Autodesk Fusion 360 part; units mm, degrees
(part 5 of 11)
  line L3350 (-0.0459, -214.2627) -> (-0.0798, -214.2989)
  line L3351 (-0.0798, -214.2989) -> (-0.1133, -214.3397)
  line L3352 (-0.1133, -214.3397) -> (-0.1441, -214.3827)
  line L3353 (-0.1441, -214.3827) -> (-0.172, -214.4275)
  line L3354 (-0.172, -214.4275) -> (-0.1969, -214.4741)
  line L3355 (-0.1969, -214.4741) -> (-0.2187, -214.5222)
  line L3356 (-0.2187, -214.5222) -> (-0.2373, -214.5717)
  line L3357 (-0.2373, -214.5717) -> (-0.2526, -214.6222)
  line L3358 (-0.2526, -214.6222) -> (-0.2646, -214.6736)
  line L3359 (-0.2646, -214.6736) -> (-0.2732, -214.7258)
  line L3360 (-0.2732, -214.7258) -> (-0.2786, -214.7804)
  line L3361 (-0.2786, -214.7804) -> (-0.28, -214.8985)
  line L3362 (-0.28, -214.8985) -> (-0.28, -218.4997)
  line L3363 (-0.28, -218.4997) -> (-0.28, -219.4997)
  arc A210 (-0.28, -219.4997) -> (0.42, -220.1997) centre (0.42, -219.4997) ccw
  line L3364 (0.42, -220.1997) -> (1.42, -220.1997)
  line L3365 (1.42, -220.1997) -> (5.0918, -220.1997)
  line L3366 (5.0918, -220.1997) -> (5.1413, -220.198)
  line L3367 (5.1413, -220.198) -> (5.1939, -220.1929)
  line L3368 (5.1939, -220.1929) -> (5.246, -220.1843)
  line L3369 (5.246, -220.1843) -> (5.2975, -220.1723)
  line L3370 (5.2975, -220.1723) -> (5.348, -220.1569)
  line L3371 (5.348, -220.1569) -> (5.3974, -220.1383)
  line L3372 (5.3974, -220.1383) -> (5.4455, -220.1165)
  line L3373 (5.4455, -220.1165) -> (5.4921, -220.0916)
  line L3374 (5.4921, -220.0916) -> (5.537, -220.0637)
  line L3375 (5.537, -220.0637) -> (5.5799, -220.033)
  line L3376 (5.5799, -220.033) -> (5.6207, -219.9995)
  line L3377 (5.6207, -219.9995) -> (5.6569, -219.9656)
  line L3378 (5.6569, -219.9656) -> (6.94, -218.6825)
  arc A211 (6.94, -218.6825) -> (6.6572, -217.9997) centre (6.6572, -218.3997) ccw
  line L3379 (6.6572, -217.9997) -> (4.62, -217.9997)
  line L3380 (4.62, -217.9997) -> (4.62, -216.6432)
  line L3381 (4.62, -216.6432) -> (7.1635, -214.0997)
  line L3382 (7.1635, -214.0997) -> (9.7981, -214.0997)
  line L3383 (9.7981, -214.0997) -> (9.9208, -213.977)
  line L3384 (9.9208, -213.977) -> (10.0448, -214.0997)
  line L3385 (10.0448, -214.0997) -> (12.6765, -214.0997)
  line L3386 (12.6765, -214.0997) -> (15.22, -216.6432)
  line L3387 (15.22, -216.6432) -> (15.22, -217.9997)
  line L3388 (15.22, -217.9997) -> (13.1828, -217.9997)
  arc A212 (13.1828, -217.9997) -> (12.9, -218.6825) centre (13.1828, -218.3997) ccw
  line L3389 (12.9, -218.6825) -> (14.1831, -219.9656)
  line L3390 (14.1831, -219.9656) -> (14.2193, -219.9995)
  line L3391 (14.2193, -219.9995) -> (14.2601, -220.033)
  line L3392 (14.2601, -220.033) -> (14.303, -220.0637)
  line L3393 (14.303, -220.0637) -> (14.3479, -220.0916)
  line L3394 (14.3479, -220.0916) -> (14.3945, -220.1165)
  line L3395 (14.3945, -220.1165) -> (14.4426, -220.1383)
  line L3396 (14.4426, -220.1383) -> (14.492, -220.1569)
  line L3397 (14.492, -220.1569) -> (14.5425, -220.1723)
  line L3398 (14.5425, -220.1723) -> (14.594, -220.1843)
  line L3399 (14.594, -220.1843) -> (14.6461, -220.1929)
  line L3400 (14.6461, -220.1929) -> (14.6987, -220.198)
  line L3401 (14.6987, -220.198) -> (14.7482, -220.1997)
  line L3402 (14.7482, -220.1997) -> (18.42, -220.1997)
  line L3403 (18.42, -220.1997) -> (19.42, -220.1997)
  arc A213 (19.42, -220.1997) -> (20.12, -219.4997) centre (19.42, -219.4997) ccw
  line L3404 (20.12, -219.4997) -> (20.12, -218.4997)
  line L3405 (20.12, -218.4997) -> (20.12, -214.8278)
  line L3406 (20.12, -214.8278) -> (20.1184, -214.7783)
  line L3407 (20.1184, -214.7783) -> (20.1132, -214.7258)
  line L3408 (20.1132, -214.7258) -> (20.1046, -214.6736)
  line L3409 (20.1046, -214.6736) -> (20.0926, -214.6222)
  line L3410 (20.0926, -214.6222) -> (20.0773, -214.5717)
  line L3411 (20.0773, -214.5717) -> (20.0587, -214.5222)
  line L3412 (20.0587, -214.5222) -> (20.0369, -214.4741)
  line L3413 (20.0369, -214.4741) -> (20.012, -214.4275)
  line L3414 (20.012, -214.4275) -> (19.9841, -214.3827)
  line L3415 (19.9841, -214.3827) -> (19.9533, -214.3397)
  line L3416 (19.9533, -214.3397) -> (19.9198, -214.2989)
  line L3417 (19.9198, -214.2989) -> (19.8859, -214.2627)
  line L3418 (19.8859, -214.2627) -> (18.6028, -212.9797)
  arc A214 (18.6028, -212.9797) -> (17.92, -213.2625) centre (18.32, -213.2625) ccw
  line L3419 (17.92, -213.2625) -> (17.92, -215.2997)
  line L3420 (17.92, -215.2997) -> (16.5635, -215.2997)
  line L3421 (16.5635, -215.2997) -> (14.02, -212.7562)
  line L3422 (14.02, -212.7562) -> (14.02, -210.1167)
  line L3423 (14.02, -210.1167) -> (13.903, -209.9997)
  line L3424 (13.903, -209.9997) -> (14.02, -209.8826)
  line L3425 (14.02, -209.8826) -> (14.02, -207.2432)
  line L3426 (14.02, -207.2432) -> (16.5635, -204.6997)
  line L3427 (16.5635, -204.6997) -> (17.92, -204.6997)
  line L3428 (17.92, -204.6997) -> (17.92, -206.7368)
  arc A215 (17.92, -206.7368) -> (18.6028, -207.0197) centre (18.32, -206.7368) ccw
  line L3429 (18.6028, -207.0197) -> (19.8859, -205.7366)
  line L3430 (19.8859, -205.7366) -> (19.9198, -205.7004)
  line L3431 (19.9198, -205.7004) -> (19.9533, -205.6596)
  line L3432 (19.9533, -205.6596) -> (19.9841, -205.6166)
  line L3433 (19.9841, -205.6166) -> (20.012, -205.5718)
  line L3434 (20.012, -205.5718) -> (20.0369, -205.5252)
  line L3435 (20.0369, -205.5252) -> (20.0587, -205.4771)
  line L3436 (20.0587, -205.4771) -> (20.0773, -205.4277)
  line L3437 (20.0773, -205.4277) -> (20.0926, -205.3771)
  line L3438 (20.0926, -205.3771) -> (20.1046, -205.3257)
  line L3439 (20.1046, -205.3257) -> (20.1132, -205.2736)
  line L3440 (20.1132, -205.2736) -> (20.1186, -205.2189)
  line L3441 (20.1186, -205.2189) -> (20.12, -205.1009)
  line L3442 (20.12, -205.1009) -> (20.12, -194.8985)
  line L3443 (20.12, -194.8985) -> (20.1186, -194.7804)
  line L3444 (20.1186, -194.7804) -> (20.1132, -194.7258)
  line L3445 (20.1132, -194.7258) -> (20.1046, -194.6736)
  line L3446 (20.1046, -194.6736) -> (20.0926, -194.6222)
  line L3447 (20.0926, -194.6222) -> (20.0773, -194.5717)
  line L3448 (20.0773, -194.5717) -> (20.0587, -194.5222)
  line L3449 (20.0587, -194.5222) -> (20.0369, -194.4741)
  line L3450 (20.0369, -194.4741) -> (20.012, -194.4275)
  line L3451 (20.012, -194.4275) -> (19.9841, -194.3827)
  line L3452 (19.9841, -194.3827) -> (19.9533, -194.3397)
  line L3453 (19.9533, -194.3397) -> (19.9198, -194.2989)
  line L3454 (19.9198, -194.2989) -> (19.8859, -194.2627)
  line L3455 (19.8859, -194.2627) -> (18.6028, -192.9797)
  arc A216 (18.6028, -192.9797) -> (17.92, -193.2625) centre (18.32, -193.2625) ccw
  line L3456 (17.92, -193.2625) -> (17.92, -195.2997)
  line L3457 (17.92, -195.2997) -> (16.5635, -195.2997)
  line L3458 (16.5635, -195.2997) -> (14.02, -192.7562)
  line L3459 (14.02, -192.7562) -> (14.02, -190.1167)
  line L3460 (14.02, -190.1167) -> (13.903, -189.9997)
  line L3461 (13.903, -189.9997) -> (14.02, -189.8826)
  line L3462 (14.02, -189.8826) -> (14.02, -187.2432)
  line L3463 (14.02, -187.2432) -> (16.5635, -184.6997)
  line L3464 (16.5635, -184.6997) -> (17.92, -184.6997)
  line L3465 (17.92, -184.6997) -> (17.92, -186.7368)
  arc A217 (17.92, -186.7368) -> (18.6028, -187.0197) centre (18.32, -186.7368) ccw
  line L3466 (18.6028, -187.0197) -> (19.8859, -185.7366)
  line L3467 (19.8859, -185.7366) -> (19.9198, -185.7004)
  line L3468 (19.9198, -185.7004) -> (19.9533, -185.6596)
  line L3469 (19.9533, -185.6596) -> (19.9841, -185.6166)
  line L3470 (19.9841, -185.6166) -> (20.012, -185.5718)
  line L3471 (20.012, -185.5718) -> (20.0369, -185.5252)
  line L3472 (20.0369, -185.5252) -> (20.0587, -185.4771)
  line L3473 (20.0587, -185.4771) -> (20.0773, -185.4277)
  line L3474 (20.0773, -185.4277) -> (20.0926, -185.3771)
  line L3475 (20.0926, -185.3771) -> (20.1046, -185.3257)
  line L3476 (20.1046, -185.3257) -> (20.1132, -185.2736)
  line L3477 (20.1132, -185.2736) -> (20.1186, -185.2189)
  line L3478 (20.1186, -185.2189) -> (20.12, -185.1009)
  line L3479 (20.12, -185.1009) -> (20.12, -174.8985)
  line L3480 (20.12, -174.8985) -> (20.1186, -174.7804)
  line L3481 (20.1186, -174.7804) -> (20.1132, -174.7258)
  line L3482 (20.1132, -174.7258) -> (20.1046, -174.6736)
  line L3483 (20.1046, -174.6736) -> (20.0926, -174.6222)
  line L3484 (20.0926, -174.6222) -> (20.0773, -174.5717)
  line L3485 (20.0773, -174.5717) -> (20.0587, -174.5222)
  line L3486 (20.0587, -174.5222) -> (20.0369, -174.4741)
  line L3487 (20.0369, -174.4741) -> (20.012, -174.4275)
  line L3488 (20.012, -174.4275) -> (19.9841, -174.3827)
  line L3489 (19.9841, -174.3827) -> (19.9533, -174.3397)
  line L3490 (19.9533, -174.3397) -> (19.9198, -174.2989)
  line L3491 (19.9198, -174.2989) -> (19.8859, -174.2627)
  line L3492 (19.8859, -174.2627) -> (18.6028, -172.9797)
  arc A218 (18.6028, -172.9797) -> (17.92, -173.2625) centre (18.32, -173.2625) ccw
  line L3493 (17.92, -173.2625) -> (17.92, -175.2997)
  line L3494 (17.92, -175.2997) -> (16.5635, -175.2997)
  line L3495 (16.5635, -175.2997) -> (14.02, -172.7562)
  line L3496 (14.02, -172.7562) -> (14.02, -170.1167)
  line L3497 (14.02, -170.1167) -> (13.903, -169.9997)
  line L3498 (13.903, -169.9997) -> (14.02, -169.8826)
  line L3499 (14.02, -169.8826) -> (14.02, -167.2432)
  line L3500 (14.02, -167.2432) -> (16.5635, -164.6997)
  line L3501 (16.5635, -164.6997) -> (17.92, -164.6997)
  line L3502 (17.92, -164.6997) -> (17.92, -166.7368)
  arc A219 (17.92, -166.7368) -> (18.6028, -167.0197) centre (18.32, -166.7368) ccw
  line L3503 (18.6028, -167.0197) -> (19.8859, -165.7366)
  line L3504 (19.8859, -165.7366) -> (19.9198, -165.7004)
  line L3505 (19.9198, -165.7004) -> (19.9533, -165.6596)
  line L3506 (19.9533, -165.6596) -> (19.9841, -165.6166)
  line L3507 (19.9841, -165.6166) -> (20.012, -165.5718)
  line L3508 (20.012, -165.5718) -> (20.0369, -165.5252)
  line L3509 (20.0369, -165.5252) -> (20.0587, -165.4771)
  line L3510 (20.0587, -165.4771) -> (20.0773, -165.4277)
  line L3511 (20.0773, -165.4277) -> (20.0926, -165.3771)
  line L3512 (20.0926, -165.3771) -> (20.1046, -165.3257)
  line L3513 (20.1046, -165.3257) -> (20.1132, -165.2736)
  line L3514 (20.1132, -165.2736) -> (20.1186, -165.2189)
  line L3515 (20.1186, -165.2189) -> (20.12, -165.1009)
  line L3516 (20.12, -165.1009) -> (20.12, -154.8985)
  line L3517 (20.12, -154.8985) -> (20.1186, -154.7804)
  line L3518 (20.1186, -154.7804) -> (20.1132, -154.7258)
  line L3519 (20.1132, -154.7258) -> (20.1046, -154.6736)
  line L3520 (20.1046, -154.6736) -> (20.0926, -154.6222)
  line L3521 (20.0926, -154.6222) -> (20.0773, -154.5717)
  line L3522 (20.0773, -154.5717) -> (20.0587, -154.5222)
  line L3523 (20.0587, -154.5222) -> (20.0369, -154.4741)
  line L3524 (20.0369, -154.4741) -> (20.012, -154.4275)
  line L3525 (20.012, -154.4275) -> (19.9841, -154.3827)
  line L3526 (19.9841, -154.3827) -> (19.9533, -154.3397)
  line L3527 (19.9533, -154.3397) -> (19.9198, -154.2989)
  line L3528 (19.9198, -154.2989) -> (19.8859, -154.2627)
  line L3529 (19.8859, -154.2627) -> (18.6028, -152.9797)
  arc A220 (18.6028, -152.9797) -> (17.92, -153.2625) centre (18.32, -153.2625) ccw
  line L3530 (17.92, -153.2625) -> (17.92, -155.2997)
  line L3531 (17.92, -155.2997) -> (16.5635, -155.2997)
  line L3532 (16.5635, -155.2997) -> (14.02, -152.7562)
  line L3533 (14.02, -152.7562) -> (14.02, -150.1167)
  line L3534 (14.02, -150.1167) -> (13.903, -149.9997)
  line L3535 (13.903, -149.9997) -> (14.02, -149.8826)
  line L3536 (14.02, -149.8826) -> (14.02, -147.2432)
  line L3537 (14.02, -147.2432) -> (16.5635, -144.6997)
  line L3538 (16.5635, -144.6997) -> (17.92, -144.6997)
  line L3539 (17.92, -144.6997) -> (17.92, -146.7368)
  arc A221 (17.92, -146.7368) -> (18.6028, -147.0197) centre (18.32, -146.7368) ccw
  line L3540 (18.6028, -147.0197) -> (19.8859, -145.7366)
  line L3541 (19.8859, -145.7366) -> (19.9198, -145.7004)
  line L3542 (19.9198, -145.7004) -> (19.9533, -145.6596)
  line L3543 (19.9533, -145.6596) -> (19.9841, -145.6166)
  line L3544 (19.9841, -145.6166) -> (20.012, -145.5718)
  line L3545 (20.012, -145.5718) -> (20.0369, -145.5252)
  line L3546 (20.0369, -145.5252) -> (20.0587, -145.4771)
  line L3547 (20.0587, -145.4771) -> (20.0773, -145.4277)
  line L3548 (20.0773, -145.4277) -> (20.0926, -145.3771)
  line L3549 (20.0926, -145.3771) -> (20.1046, -145.3257)
  line L3550 (20.1046, -145.3257) -> (20.1132, -145.2736)
  line L3551 (20.1132, -145.2736) -> (20.1184, -145.221)
  line L3552 (20.1184, -145.221) -> (20.12, -145.1715)
  line L3553 (20.12, -145.1715) -> (20.12, -141.4997)
  line L3554 (20.12, -141.4997) -> (20.12, -140.4997)
  arc A222 (20.12, -140.4997) -> (19.42, -139.7997) centre (19.42, -140.4997) ccw
  line L3555 (19.42, -139.7997) -> (18.42, -139.7997)
  line L3556 (18.42, -139.7997) -> (14.7482, -139.7997)
  line L3557 (14.7482, -139.7997) -> (14.6987, -139.8013)
  line L3558 (14.6987, -139.8013) -> (14.6461, -139.8065)
  line L3559 (14.6461, -139.8065) -> (14.594, -139.8151)
  line L3560 (14.594, -139.8151) -> (14.5425, -139.8271)
  line L3561 (14.5425, -139.8271) -> (14.492, -139.8424)
  line L3562 (14.492, -139.8424) -> (14.4426, -139.861)
  line L3563 (14.4426, -139.861) -> (14.3945, -139.8828)
  line L3564 (14.3945, -139.8828) -> (14.3479, -139.9077)
  line L3565 (14.3479, -139.9077) -> (14.303, -139.9356)
  line L3566 (14.303, -139.9356) -> (14.2601, -139.9663)
  line L3567 (14.2601, -139.9663) -> (14.2193, -139.9999)
  line L3568 (14.2193, -139.9999) -> (14.1831, -140.0337)
  line L3569 (14.1831, -140.0337) -> (12.9, -141.3168)
  arc A223 (12.9, -141.3168) -> (13.1828, -141.9997) centre (13.1828, -141.5997) ccw
  line L3570 (13.1828, -141.9997) -> (15.22, -141.9997)
  line L3571 (15.22, -141.9997) -> (15.22, -143.3562)
  line L3572 (15.22, -143.3562) -> (12.6765, -145.8997)
  line L3573 (12.6765, -145.8997) -> (10.0448, -145.8997)
  line L3574 (10.0448, -145.8997) -> (9.9208, -146.0223)
  line L3575 (9.9208, -146.0223) -> (9.7981, -145.8997)
  line L3576 (9.7981, -145.8997) -> (7.1635, -145.8997)
  line L3577 (7.1635, -145.8997) -> (4.62, -143.3562)
  line L3578 (4.62, -143.3562) -> (4.62, -141.9997)
  line L3579 (4.62, -141.9997) -> (6.6572, -141.9997)
  arc A224 (6.6572, -141.9997) -> (6.94, -141.3168) centre (6.6572, -141.5997) ccw
  line L3580 (6.94, -141.3168) -> (5.6569, -140.0337)
  line L3581 (5.6569, -140.0337) -> (5.6207, -139.9999)
  line L3582 (5.6207, -139.9999) -> (5.5799, -139.9663)
  line L3583 (5.5799, -139.9663) -> (5.537, -139.9356)
  line L3584 (5.537, -139.9356) -> (5.4921, -139.9077)
  line L3585 (5.4921, -139.9077) -> (5.4455, -139.8828)
  line L3586 (5.4455, -139.8828) -> (5.3974, -139.861)
  line L3587 (5.3974, -139.861) -> (5.348, -139.8424)
  line L3588 (5.348, -139.8424) -> (5.2975, -139.8271)
  line L3589 (5.2975, -139.8271) -> (5.246, -139.8151)
  line L3590 (5.246, -139.8151) -> (5.1939, -139.8065)
  line L3591 (5.1939, -139.8065) -> (5.1413, -139.8013)
  line L3592 (5.1413, -139.8013) -> (5.0918, -139.7997)
  line L3593 (5.0918, -139.7997) -> (1.42, -139.7997)
  line L3594 (1.42, -139.7997) -> (0.42, -139.7997)
  arc A225 (0.42, -139.7997) -> (-0.28, -140.4997) centre (0.42, -140.4997) ccw
  line L3595 (-0.28, -140.4997) -> (-0.28, -141.4997)
  line L3596 (-0.28, -141.4997) -> (-0.28, -145.1009)
  line L3597 (-0.28, -145.1009) -> (-0.2786, -145.2189)
  line L3598 (16.0765, -157.4997) -> (17.92, -157.4997)
  line L3599 (17.92, -157.4997) -> (17.92, -162.4997)
  line L3600 (17.92, -162.4997) -> (16.0765, -162.4997)
  line L3601 (16.0765, -162.4997) -> (12.6765, -165.8997)
  line L3602 (12.6765, -165.8997) -> (10.0441, -165.8997)
  line L3603 (10.0441, -165.8997) -> (9.92, -166.0238)
  line L3604 (9.92, -166.0238) -> (9.7959, -165.8997)
  line L3605 (9.7959, -165.8997) -> (7.1635, -165.8997)
  line L3606 (7.1635, -165.8997) -> (3.7635, -162.4997)
  line L3607 (3.7635, -162.4997) -> (1.92, -162.4997)
  line L3608 (1.92, -162.4997) -> (1.92, -157.4997)
  line L3609 (1.92, -157.4997) -> (3.7635, -157.4997)
  line L3610 (3.7635, -157.4997) -> (7.1635, -154.0997)
  line L3611 (7.1635, -154.0997) -> (9.7959, -154.0997)
  line L3612 (9.7959, -154.0997) -> (9.92, -153.9755)
  line L3613 (9.92, -153.9755) -> (10.0441, -154.0997)
  line L3614 (10.0441, -154.0997) -> (12.6765, -154.0997)
  line L3615 (12.6765, -154.0997) -> (16.0765, -157.4997)
  line L3616 (9.92, -173.9755) -> (10.0441, -174.0997)
  line L3617 (10.0441, -174.0997) -> (12.6765, -174.0997)
  line L3618 (12.6765, -174.0997) -> (16.0765, -177.4997)
  line L3619 (16.0765, -177.4997) -> (17.92, -177.4997)
  line L3620 (17.92, -177.4997) -> (17.92, -182.4997)
  line L3621 (17.92, -182.4997) -> (16.0765, -182.4997)
  line L3622 (16.0765, -182.4997) -> (12.6765, -185.8997)
  line L3623 (12.6765, -185.8997) -> (10.0441, -185.8997)
  line L3624 (10.0441, -185.8997) -> (9.92, -186.0238)
  line L3625 (9.92, -186.0238) -> (9.7959, -185.8997)
  line L3626 (9.7959, -185.8997) -> (7.1635, -185.8997)
  line L3627 (7.1635, -185.8997) -> (3.7635, -182.4997)
  line L3628 (3.7635, -182.4997) -> (1.92, -182.4997)
  line L3629 (1.92, -182.4997) -> (1.92, -177.4997)
  line L3630 (1.92, -177.4997) -> (3.7635, -177.4997)
  line L3631 (3.7635, -177.4997) -> (7.1635, -174.0997)
  line L3632 (7.1635, -174.0997) -> (9.7959, -174.0997)
  line L3633 (9.7959, -174.0997) -> (9.92, -173.9755)
  line L3634 (9.92, -193.9755) -> (10.0441, -194.0997)
  line L3635 (10.0441, -194.0997) -> (12.6765, -194.0997)
  line L3636 (12.6765, -194.0997) -> (16.0765, -197.4997)
  line L3637 (16.0765, -197.4997) -> (17.92, -197.4997)
  line L3638 (17.92, -197.4997) -> (17.92, -202.4997)
  line L3639 (17.92, -202.4997) -> (16.0765, -202.4997)
  line L3640 (16.0765, -202.4997) -> (12.6765, -205.8997)
  line L3641 (12.6765, -205.8997) -> (10.0441, -205.8997)
  line L3642 (10.0441, -205.8997) -> (9.92, -206.0238)
  line L3643 (9.92, -206.0238) -> (9.7959, -205.8997)
  line L3644 (9.7959, -205.8997) -> (7.1635, -205.8997)
  line L3645 (7.1635, -205.8997) -> (3.7635, -202.4997)
  line L3646 (3.7635, -202.4997) -> (1.92, -202.4997)
  line L3647 (1.92, -202.4997) -> (1.92, -197.4997)
  line L3648 (1.92, -197.4997) -> (3.7635, -197.4997)
  line L3649 (3.7635, -197.4997) -> (7.1635, -194.0997)
  line L3650 (7.1635, -194.0997) -> (9.7959, -194.0997)
  line L3651 (9.7959, -194.0997) -> (9.92, -193.9755)
  point P0 (-0.08, -109.9997)
  point P1 (9.92, -109.9997)
  point P2 (9.92, -179.9997)
  point P3 (9.92, -39.9997)
  dimension "d7" = 0.2
  dimension "d8" = 0.2
  dimension "d9" = 0.2
  dimension "d10" = 0.2
  dimension "d11" = 0.2
  dimension "d12" = 0.2
  dimension "d13" = 0.2
  dimension "d14" = 0.2
  dimension "d15" = 0.2
  dimension "d16" = 0.2
  dimension "d17" = 0.2